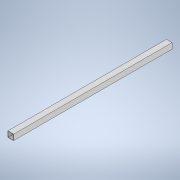
# Autodesk Inventor part: 1x1 Stock 28in
Saved by Autodesk Inventor 2020 (Build 240168000, 168)
## iProperties
Created: 2020-01-14
Part Number: 1x1 Stock 28in
Material: Generic
Document SubType Name: Modeling
Designer: aidan
Density: 1 g/cm^3
Appearance: Default
Author: aidan
Autodesk Inventor part; units mm, degrees
ref_plane "YZ Plane" through (0, 0, 0) normal (1, 0, 0) x (0, 1, 0)
ref_plane "XZ Plane" through (0, 0, 0) normal (0, 1, 0) x (-1, 0, 0)
ref_plane "XY Plane" through (0, 0, 0) normal (0, 0, 1) x (1, 0, 0)
sketch "Sketch1" plane through (0, 0, 0) normal (0, 0, 1) x (1, 0, 0)
  line L0 (-14.0074, 10.2243) -> (11.3926, 10.2243)
  line L1 (11.3926, 10.2243) -> (11.3926, -15.1757)
  line L2 (11.3926, -15.1757) -> (-14.0074, -15.1757)
  line L3 (-14.0074, -15.1757) -> (-14.0074, 10.2243)
  line L4 (10.1226, 8.9543) -> (-12.7374, 8.9543)
  line L5 (-12.7374, 8.9543) -> (-12.7374, -13.9057)
  line L6 (-12.7374, -13.9057) -> (10.1226, -13.9057)
  line L7 (10.1226, -13.9057) -> (10.1226, 8.9543)
  point P0 (0, 0)
  dimension "d0" = 25.4
  dimension "d1" = 1.27
  constraints: 16 end point, 4 parallel, 3 perpendicular, 1 horizontal, 3 other
  measures "d0" distance of L0.start L0.end
  measures "d1" distance between parallel lines of L0 L4
extrude "Extrusion1" add sketch "Sketch1" along normal blind 711.2
body "Solid1"
